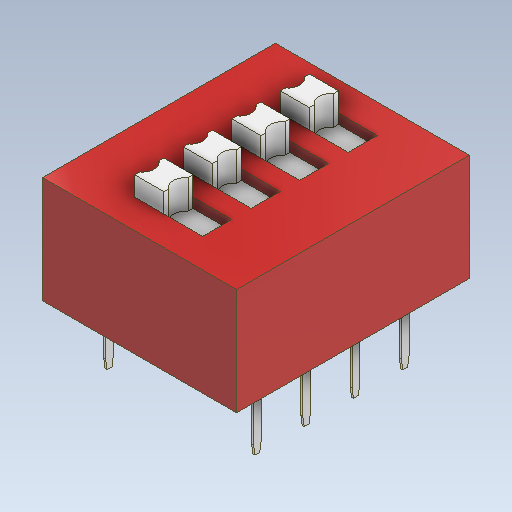
# Autodesk Inventor part: Dip_switch_4
Saved by Autodesk Inventor 2020 (Build 240168000, 168)
## iProperties
Created: 2019-12-30
Part Number: Dip_switch_4
Material: Polypropylene
Document SubType Name: Modeling
Designer: ermoz
Density: 0.899 g/cm^3
Appearance: Smooth - Ash
Mass: 0.595132 g
Surface Area: 7.29198 cm^2
Volume: 0.661993 cm^3
Author: ermoz
Autodesk Inventor part; units mm, degrees
ref_plane "YZ Plane" through (0, 0, 0) normal (1, 0, 0) x (0, 1, 0)
ref_plane "XZ Plane" through (0, 0, 0) normal (0, 1, 0) x (-1, 0, 0)
ref_plane "XY Plane" through (0, 0, 0) normal (0, 0, 1) x (1, 0, 0)
sketch "Sketch1" plane through (0, 0, 0) normal (0, 1, 0) x (-1, 0, 0)
  line L0 (5, 7.25) -> (-5, 7.25)
  line L1 (-5, 7.25) -> (-5, -7.25)
  line L2 (-5, -7.25) -> (5, -7.25)
  line L3 (5, -7.25) -> (5, 7.25)
  line L4 (5, 7.25) -> (-5, -7.25) construction
  line L5 (-5, 7.25) -> (5, -7.25) construction
  point P0 (0, 0)
  dimension "d0" = 10
  dimension "d1" = 14.5
  constraints: 12 end point, 2 midpoint, 2 parallel, 1 horizontal, 1 perpendicular
  measures "d0" distance of L2.end L1.end
  measures "d1" distance of L1.end L0.end
extrude "Extrusion1" add sketch "Sketch1" along normal blind 5.5
sketch "Sketch2" plane through (0, 5.5, 0) normal (0, 1, 0) x (1, 0, 0)
  line L0 (-1.75, 0.75) -> (1.75, 0.75)
  line L1 (1.75, 0.75) -> (1.75, -0.75)
  line L2 (1.75, -0.75) -> (-1.75, -0.75)
  line L3 (-1.75, -0.75) -> (-1.75, 0.75)
  line L4 (-1.75, 0.75) -> (1.75, -0.75) construction
  line L5 (1.75, 0.75) -> (-1.75, -0.75) construction
  line L6 (0, -0.75) -> (0, -1.75)
  line L7 (0, -1.75) -> (0, -2.5)
  line L8 (-1.75, -1.75) -> (1.75, -1.75)
  line L9 (1.75, -1.75) -> (1.75, -3.25)
  line L10 (1.75, -3.25) -> (-1.75, -3.25)
  line L11 (-1.75, -3.25) -> (-1.75, -1.75)
  line L12 (-1.75, -1.75) -> (1.75, -3.25) construction
  line L13 (1.75, -1.75) -> (-1.75, -3.25) construction
  line L14 (0, -3.25) -> (0, -5)
  line L15 (-1.75, -4.25) -> (1.75, -4.25)
  line L16 (1.75, -4.25) -> (1.75, -5.75)
  line L17 (1.75, -5.75) -> (-1.75, -5.75)
  line L18 (-1.75, -5.75) -> (-1.75, -4.25)
  line L19 (-1.75, -4.25) -> (1.75, -5.75) construction
  line L20 (1.75, -4.25) -> (-1.75, -5.75) construction
  line L21 (0, 0) -> (3.2691, 0)
  line L22 (-1.75, 1.75) -> (1.75, 1.75)
  line L23 (1.75, 1.75) -> (1.75, 3.25)
  line L24 (1.75, 3.25) -> (-1.75, 3.25)
  line L25 (-1.75, 3.25) -> (-1.75, 1.75)
  line L26 (-1.75, 4.25) -> (1.75, 4.25)
  line L27 (1.75, 4.25) -> (1.75, 5.75)
  line L28 (1.75, 5.75) -> (-1.75, 5.75)
  line L29 (-1.75, 5.75) -> (-1.75, 4.25)
  dimension "d4" = 3.5
  dimension "d5" = 1.5
  dimension "d6" = 1
  dimension "d7" = 0.75
  dimension "d8" = 3.5
  dimension "d9" = 1.5
  dimension "d10" = 1.75
  dimension "d11" = 3.5
  dimension "d12" = 1.5
  constraints: 60 end point, 8 midpoint, 8 symmetric about line, 6 parallel, 4 horizontal, 3 perpendicular, 3 vertical
  measures "d4" distance of L1.end L2.end
  measures "d5" distance of L0.end L1.end
  measures "d6" distance of L6.start L6.end
  measures "d7" distance of L6.end L7.end
  measures "d8" distance of L9.end L10.end
  measures "d9" distance of L8.end L9.end
  measures "d10" distance of L14.start L14.end
  measures "d11" distance of L16.end L17.end
  measures "d12" distance of L15.end L16.end
extrude "Extrusion2" cut sketch "Sketch2" against normal blind 2
extrude "Extrusion3" add sketch "Sketch2" against normal blind 2 separate body
sketch "Sketch3" plane through (0, 5.5, 0) normal (0, 1, 0) x (1, 0, 0)
  line L0 (1.75, 5.75) -> (1.75, 4.25) projected
  line L1 (1.75, -5.75) -> (-1.75, -5.75) projected
  line L2 (1.75, 5.75) -> (-1.75, 5.75)
  line L3 (-1.75, 5.75) -> (-1.75, -5.75)
  line L4 (-1.75, -5.75) -> (1.75, -5.75)
  line L5 (1.75, -5.75) -> (1.75, 5.75)
  point P0 (0, 0)
  constraints: 8 end point, 2 parallel, 1 horizontal, 1 perpendicular
extrude "Extrusion4" cut sketch "Sketch3" against normal blind 0.5 bodies 2
sketch "Sketch4" plane through (0, 5, 0) normal (0, 1, 0) x (1, 0, 0)
  line L0 (-1.75, 5.75) -> (1.75, 5.75) projected
  line L1 (1.75, 4.25) -> (-1.75, 4.25) projected
  line L2 (-1.75, 5.75) -> (-0.25, 5.75)
  line L3 (-0.25, 4.25) -> (-1.75, 4.25)
  line L4 (1.75, 1.75) -> (-1.75, 1.75) projected
  line L5 (-1.75, 3.25) -> (-0.25, 3.25)
  line L6 (-0.25, 1.75) -> (-1.75, 1.75)
  line L7 (-1.75, 0.75) -> (1.75, 0.75) projected
  line L8 (1.75, -0.75) -> (-1.75, -0.75) projected
  line L9 (-1.75, 0.75) -> (-0.25, 0.75)
  line L10 (-0.25, -0.75) -> (-1.75, -0.75)
  line L11 (-1.75, -0.75) -> (-1.75, 0.75)
  line L12 (-1.75, -1.75) -> (1.75, -1.75) projected
  line L13 (1.75, -3.25) -> (-1.75, -3.25) projected
  line L14 (-1.75, -1.75) -> (-0.25, -1.75)
  line L15 (-0.25, -1.75) -> (-0.25, -3.25)
  line L16 (-0.25, -3.25) -> (-1.75, -3.25)
  line L17 (-1.75, -3.25) -> (-1.75, -1.75)
  line L18 (-1.75, -4.25) -> (1.75, -4.25) projected
  line L19 (1.75, -5.75) -> (-1.75, -5.75) projected
  line L20 (-1.75, -4.25) -> (-0.25, -4.25)
  line L21 (-0.25, -4.25) -> (-0.25, -5.75)
  line L22 (-0.25, -5.75) -> (-1.75, -5.75)
  line L23 (-1.75, -5.75) -> (-1.75, -4.25)
  line L24 (-1.75, 0) -> (-1.5, 0)
  line L25 (-0.25, 0) -> (-0.5, 0)
  line L26 (-1, 5.75) -> (-1, 5.5)
  line L27 (-1, 4.25) -> (-1, 4.5)
  line L28 (-1.75, 4.25) -> (-1.75, 5.75) projected
  arc A0 (-1.75, 4.5) -> (-1.75, 5.5) centre (-2.125, 5) ccw
  line L29 (-1, 1.75) -> (-1, 2)
  line L30 (-1.75, 3.25) -> (1.75, 3.25) projected
  line L31 (-1, 3.25) -> (-1, 3)
  line L32 (-1.75, 1.75) -> (-1.75, 3.25) projected
  line L33 (-1.75, 3) -> (-1.75, 2)
  arc A1 (-1.75, 2) -> (-1.75, 3) centre (-2.125, 2.5) ccw
  line L34 (-1, 0.75) -> (-1, 0.5)
  line L35 (-1, -0.75) -> (-1, -0.5)
  arc A2 (-1.75, -0.5) -> (-1.75, 0.5) centre (-2.125, 0) ccw
  arc A3 (-0.25, 5.5) -> (-0.25, 4.5) centre (0.125, 5) ccw
  arc A4 (-0.25, 3) -> (-0.25, 2) centre (0.125, 2.5) ccw
  arc A5 (-0.25, 0.5) -> (-0.25, -0.5) centre (0.125, 0) ccw
  line L36 (-1.2232, 0) -> (-0.6567, 0)
  arc A6 (-1.75, -5.5) -> (-1.75, -4.5) centre (-2.125, -5) ccw
  arc A7 (-1.75, -3) -> (-1.75, -2) centre (-2.125, -2.5) ccw
  arc A8 (-1.75, -0.5) -> (-1.75, 0.5) centre (-2.125, 0) ccw
  arc A9 (-0.25, -4.5) -> (-0.25, -5.5) centre (0.125, -5) ccw
  arc A10 (-0.25, -2) -> (-0.25, -3) centre (0.125, -2.5) ccw
  line L37 (-0.25, 5.5) -> (-0.25, 5.75)
  line L38 (-0.25, 5.75) -> (-1.75, 5.75)
  line L39 (-1.75, 5.5) -> (-1.75, 5.75)
  line L40 (-0.25, 4.5) -> (-0.25, 4.25)
  line L41 (-1.75, 4.25) -> (-0.25, 4.25)
  line L42 (-1.75, 4.25) -> (-1.75, 4.5)
  line L43 (-0.25, 3) -> (-0.25, 3.25)
  line L44 (-0.25, 3.25) -> (-1.75, 3.25)
  line L45 (-1.75, 3.25) -> (-1.75, 3)
  line L46 (-1.75, 2) -> (-1.75, 1.75)
  line L47 (-1.75, 1.75) -> (-0.25, 1.75)
  line L48 (-0.25, 2) -> (-0.25, 1.75)
  line L49 (-0.25, 1.75) -> (-1.75, 1.75)
  line L50 (-0.25, 0.5) -> (-0.25, 0.75)
  line L51 (-0.25, 0.75) -> (-1.75, 0.75)
  line L52 (-1.75, 0.75) -> (-1.75, 0.5)
  line L53 (-1.75, -5.75) -> (1.75, -5.75)
  line L54 (1.75, -4.25) -> (-1.75, -4.25)
  line L55 (-1.75, -3.25) -> (-0.25, -3.25)
  line L56 (-0.25, -1.75) -> (-1.75, -1.75)
  line L57 (-1.75, -0.75) -> (-0.25, -0.75)
  line L58 (-1.75, 0.75) -> (-1.75, -0.75)
  line L59 (-1.75, -4.25) -> (-1.75, -5.75)
  line L60 (-1.75, -1.75) -> (-1.75, -3.25)
  line L61 (-0.25, -5.5) -> (-0.25, -5.75)
  line L62 (-0.25, -4.5) -> (-0.25, -4.25)
  line L63 (-1.75, -4.25) -> (-1.75, -4.5)
  line L64 (-0.25, -3) -> (-0.25, -3.25)
  line L65 (-1.75, -3.25) -> (-1.75, -3)
  line L66 (-0.25, -2) -> (-0.25, -1.75)
  line L67 (-0.25, -0.5) -> (-0.25, -0.75)
  point P0 (0, 0)
  point P1 (-0.25, -5.5)
  point P2 (-1.75, -2)
  point P3 (-0.25, -3)
  point P4 (-0.25, -2)
  point P5 (-1.75, 0.5)
  dimension "d20" = 0.25
  dimension "d21" = 0.25
  dimension "d22" = 0.25
  dimension "d23" = 0.25
  dimension "d24" = 0.25
  dimension "d25" = 0.25
  dimension "d26" = 0.25
  dimension "d27" = 0.25
  constraints: 112 end point, 29 symmetric about line, 23 point on circle, 14 point on line, 11 centre point, 9 horizontal, 7 parallel, 6 collinear, 6 vertical, 5 midpoint, 5 perpendicular, 8 other
  measures "d20" distance of L24.start L24.end
  measures "d21" distance of L25.start L25.end
  measures "d22" distance of L26.start L26.end
  measures "d23" distance of L27.start L27.end
  measures "d24" distance of L29.start L29.end
  measures "d25" distance of L31.start L31.end
  measures "d26" distance of L34.start L34.end
  measures "d27" distance of L35.start L35.end
extrude "Extrusion5" add sketch "Sketch4" along normal blind 1.5 contours L0 L37 A3 L40 L1 L28 A0 | L4 L32 A1 L5 L43 A4 L48 | L7 L50 A5 L67 L8 L11 A2 | L12 L15 A10 L13 L17 A7 | L18 L21 A9 L19 L23 A6 bodies 2
sketch "Sketch5" plane through (0, 0, 0) normal (0, -1, 0) x (1, 0, 0)
  line L0 (0, 0) -> (1.27, 0)
  line L1 (1.27, 0) -> (3.81, 0)
  line L2 (0, 0) -> (0, -1.4789)
  line L3 (3.76, 0.2) -> (3.86, 0.2)
  line L4 (3.86, 0.2) -> (3.86, -0.2)
  line L5 (3.86, -0.2) -> (3.76, -0.2)
  line L6 (3.76, -0.2) -> (3.76, 0.2)
  line L7 (3.76, 0.2) -> (3.86, -0.2) construction
  line L8 (3.86, 0.2) -> (3.76, -0.2) construction
  line L9 (3.76, -2.34) -> (3.86, -2.34)
  line L10 (3.86, -2.34) -> (3.86, -2.74)
  line L11 (3.86, -2.74) -> (3.76, -2.74)
  line L12 (3.76, -2.74) -> (3.76, -2.34)
  line L13 (3.76, -2.34) -> (3.86, -2.74) construction
  line L14 (3.86, -2.34) -> (3.76, -2.74) construction
  line L15 (3.76, -4.88) -> (3.86, -4.88)
  line L16 (3.86, -4.88) -> (3.86, -5.28)
  line L17 (3.86, -5.28) -> (3.76, -5.28)
  line L18 (3.76, -5.28) -> (3.76, -4.88)
  line L19 (3.76, -4.88) -> (3.86, -5.28) construction
  line L20 (3.86, -4.88) -> (3.76, -5.28) construction
  line L21 (3.76, -0.2) -> (3.86, -0.2)
  line L22 (3.86, -0.2) -> (3.86, 0.2)
  line L23 (3.86, 0.2) -> (3.76, 0.2)
  line L24 (3.76, 0.2) -> (3.76, -0.2)
  line L25 (3.76, 2.34) -> (3.86, 2.34)
  line L26 (3.86, 2.34) -> (3.86, 2.74)
  line L27 (3.86, 2.74) -> (3.76, 2.74)
  line L28 (3.76, 2.74) -> (3.76, 2.34)
  line L29 (3.76, 4.88) -> (3.86, 4.88)
  line L30 (3.86, 4.88) -> (3.86, 5.28)
  line L31 (3.86, 5.28) -> (3.76, 5.28)
  line L32 (3.76, 5.28) -> (3.76, 4.88)
  line L33 (-3.76, 0.2) -> (-3.86, 0.2)
  line L34 (-3.86, 0.2) -> (-3.86, -0.2)
  line L35 (-3.86, -0.2) -> (-3.76, -0.2)
  line L36 (-3.76, -0.2) -> (-3.76, 0.2)
  line L37 (-3.76, -2.34) -> (-3.86, -2.34)
  line L38 (-3.86, -2.34) -> (-3.86, -2.74)
  line L39 (-3.86, -2.74) -> (-3.76, -2.74)
  line L40 (-3.76, -2.74) -> (-3.76, -2.34)
  line L41 (-3.76, -4.88) -> (-3.86, -4.88)
  line L42 (-3.86, -4.88) -> (-3.86, -5.28)
  line L43 (-3.86, -5.28) -> (-3.76, -5.28)
  line L44 (-3.76, -5.28) -> (-3.76, -4.88)
  line L45 (-3.76, 2.34) -> (-3.86, 2.34)
  line L46 (-3.86, 2.34) -> (-3.86, 2.74)
  line L47 (-3.86, 2.74) -> (-3.76, 2.74)
  line L48 (-3.76, 2.74) -> (-3.76, 2.34)
  line L49 (-3.76, 4.88) -> (-3.86, 4.88)
  line L50 (-3.86, 4.88) -> (-3.86, 5.28)
  line L51 (-3.86, 5.28) -> (-3.76, 5.28)
  line L52 (-3.76, 5.28) -> (-3.76, 4.88)
  dimension "d30" = 1.27
  dimension "d31" = 2.54
  dimension "d34" = 0.1
  dimension "d35" = 0.4
  dimension "d36" = 0.1
  dimension "d37" = 0.4
  dimension "d38" = 0.1
  dimension "d39" = 0.4
  constraints: 106 end point, 32 symmetric about line, 6 parallel, 4 horizontal, 3 perpendicular, 2 midpoint, 1 point on line, 1 vertical
  measures "d30" distance of L0.start L0.end
  measures "d31" distance of L0.end L1.end
  measures "d34" distance of L4.end L5.end
  measures "d35" distance of L3.end L4.end
  measures "d36" distance of L10.end L11.end
  measures "d37" distance of L9.end L10.end
  measures "d38" distance of L16.end L17.end
  measures "d39" distance of L15.end L16.end
extrude "Extrusion6" add sketch "Sketch5" along normal blind 3.5 bodies 1
chamfer "Chamfer1" distance 0.075 distance2 0.5 1 edges at (-3.81, -3.5, -5.28) measured on face at (-3.8267, -3.5, -5.0133)
chamfer "Chamfer2" distance 0.075 distance2 0.5 1 edges at (-3.81, -3.5, -2.74) measured on face at (-3.8267, -3.5, -2.4733)
chamfer "Chamfer3" distance 0.075 distance2 0.5 1 edges at (-3.81, -3.5, -0.2) measured on face at (-3.7933, -3.5, -0.0667)
chamfer "Chamfer4" distance 0.075 distance2 0.5 1 edges at (-3.81, -3.5, 2.34) measured on face at (-3.7933, -3.5, 2.4733)
chamfer "Chamfer5" distance 0.075 distance2 0.5 1 edges at (-3.81, -3.5, 4.88) measured on face at (-3.8267, -3.5, 5.1467)
chamfer "Chamfer6" distance 0.075 distance2 0.5 1 edges at (-3.81, -3.5, -4.88) measured on face at (-3.8267, -3.5, -4.9883)
chamfer "Chamfer7" distance 0.075 distance2 0.5 1 edges at (-3.81, -3.5, -2.34) measured on face at (-3.8267, -3.5, -2.4483)
chamfer "Chamfer8" distance 0.075 distance2 0.5 1 edges at (-3.81, -3.5, 0.2) measured on face at (-3.8267, -3.5, 0.0917)
chamfer "Chamfer9" distance 0.075 distance2 0.5 1 edges at (-3.81, -3.5, 2.74) measured on face at (-3.8267, -3.5, 2.6317)
chamfer "Chamfer10" distance 0.075 distance2 0.5 1 edges at (-3.81, -3.5, 5.28) measured on face at (-3.8267, -3.5, 5.1717)
chamfer "Chamfer11" distance 0.075 distance2 0.5 1 edges at (3.81, -3.5, -5.28) measured on face at (3.8267, -3.5, -5.1467)
chamfer "Chamfer12" distance 0.075 distance2 0.5 1 edges at (3.81, -3.5, -2.74) measured on face at (3.8267, -3.5, -2.6067)
chamfer "Chamfer13" distance 0.075 distance2 0.5 1 edges at (3.81, -3.5, -0.2) measured on face at (3.7933, -3.5, 0.0667)
chamfer "Chamfer14" distance 0.075 distance2 0.5 1 edges at (3.81, -3.5, 2.34) measured on face at (3.7933, -3.5, 2.6067)
chamfer "Chamfer15" distance 0.075 distance2 0.5 1 edges at (3.81, -3.5, 4.88) measured on face at (3.7933, -3.5, 5.1467)
chamfer "Chamfer16" distance 0.075 distance2 0.5 1 edges at (3.81, -3.5, 5.28) measured on face at (3.7933, -3.5, 5.1717)
chamfer "Chamfer17" distance 0.075 distance2 0.5 1 edges at (3.81, -3.5, 2.74) measured on face at (3.7933, -3.5, 2.6317)
chamfer "Chamfer18" distance 0.075 distance2 0.5 1 edges at (3.81, -3.5, 0.2) measured on face at (3.7933, -3.5, 0.0917)
chamfer "Chamfer19" distance 0.075 distance2 0.5 1 edges at (3.81, -3.5, -2.34) measured on face at (3.7933, -3.5, -2.4483)
chamfer "Chamfer20" distance 0.075 distance2 0.5 1 edges at (3.81, -3.5, -4.88) measured on face at (3.7933, -3.5, -5.0967)
sketch "Sketch7" plane through (-5, 0, 7.25) normal (0, 0, 1) x (1, 0, 0)
  line L0 (-4.1539, 9.366) -> (15.3013, 9.366)
  line L1 (15.3013, 9.366) -> (15.3013, -3.0804)
  line L2 (15.3013, -3.0804) -> (-4.1539, -3.0804)
  line L3 (-4.1539, -3.0804) -> (-4.1539, 9.366)
  point P0 (5, 0)
  constraints: 8 end point, 2 parallel, 1 horizontal, 1 perpendicular
extrude "Extrusion7" cut sketch "Sketch7" against normal blind 3 bodies 1
sketch "Sketch8" plane through (-1.75, 3.5, 5.75) normal (0, 0, 1) x (1, 0, 0)
  line L0 (-1.9166, 4.2696) -> (5.7159, 4.2696)
  line L1 (5.7159, 4.2696) -> (5.7159, -0.8935)
  line L2 (5.7159, -0.8935) -> (-1.9166, -0.8935)
  line L3 (-1.9166, -0.8935) -> (-1.9166, 4.2696)
  point P0 (1.75, -3.5)
  constraints: 8 end point, 2 parallel, 1 horizontal, 1 perpendicular
extrude "Extrusion8" cut sketch "Sketch8" against normal blind 1.5 bodies 2
sketch "Sketch9" plane through (-5, 5.5, 4.25) normal (0, 0, 1) x (1, 0, 0)
  line L0 (0, -5.5) -> (0, 0) projected
  line L1 (10, 0) -> (10, -5.5) projected
  line L2 (0, 0) -> (10, 0)
  line L3 (10, 0) -> (10, -5.5)
  line L4 (10, -5.5) -> (0, -5.5)
  line L5 (0, -5.5) -> (0, 0)
  point P0 (5, -5.5)
  constraints: 8 end point, 2 parallel, 1 horizontal, 1 perpendicular
extrude "Extrusion9" add sketch "Sketch9" along normal blind 0.5 bodies 1
sketch "Sketch10" plane through (-3.86, -3.5, 4.955) normal (-1, 0, 0) x (0, 0, 1)
  line L0 (-0.4903, 1.093) -> (1.3305, 1.093)
  line L1 (1.3305, 1.093) -> (1.3305, -0.5781)
  line L2 (1.3305, -0.5781) -> (-0.4903, -0.5781)
  line L3 (-0.4903, -0.5781) -> (-0.4903, 1.093)
  point P0 (-4.955, 3.5)
  constraints: 8 end point, 2 parallel, 1 horizontal, 1 perpendicular
extrude "Extrusion10" cut sketch "Sketch10" against normal blind 10 bodies 1
body "Solid1"
body "Solid2"
